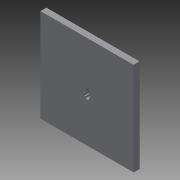
# Autodesk Inventor part: screwlockgen
Saved by Autodesk Inventor 2014 (Build 180170000, 170)
## iProperties
Created: 2014-07-13
Part Number: screwlockgen
Material: Generic
Document SubType Name: Modeling
Designer: cruiser
Density: 1 g/cm^3
Appearance: Default
Author: cruiser
Autodesk Inventor part; units mm, degrees
ref_plane "YZ Plane" through (0, 0, 0) normal (1, 0, 0) x (0, 1, 0)
ref_plane "XZ Plane" through (0, 0, 0) normal (0, 1, 0) x (-1, 0, 0)
ref_plane "XY Plane" through (0, 0, 0) normal (0, 0, 1) x (1, 0, 0)
sketch "Sketch1" plane through (0, 0, 0) normal (0, 1, 0) x (-1, 0, 0)
  line L0 (50, -50) -> (-50, -50)
  line L1 (-50, -50) -> (-50, 50)
  line L2 (-50, 50) -> (50, 50)
  line L3 (50, 50) -> (50, -50)
  line L4 (50, -50) -> (-50, 50) construction
  line L5 (-50, -50) -> (50, 50) construction
  point P0 (0, 0)
  dimension "d0" = 100
  dimension "d1" = 100
  constraints: 12 end point, 2 midpoint, 2 parallel, 1 horizontal, 1 perpendicular
  measures "d0" distance of L1.end L2.end
  measures "d1" distance of L0.end L1.end
extrude "Extrusion1" add sketch "Sketch1" along normal blind 6.35
sketch "Sketch7" plane through (0, 0, 0) normal (0, -1, 0) x (1, 0, 0)
  line L0 (1.65, -3.55) -> (-1.65, -3.55)
  line L1 (-1.65, -3.55) -> (-1.65, 3.55)
  line L2 (-1.65, 3.55) -> (1.65, 3.55)
  line L3 (1.65, 3.55) -> (1.65, -3.55)
  line L4 (1.65, -3.55) -> (-1.65, 3.55) construction
  line L5 (-1.65, -3.55) -> (1.65, 3.55) construction
  line L6 (2.75, -5.05) -> (-2.75, -5.05)
  line L7 (-2.75, -5.05) -> (-2.75, -2.05)
  line L8 (-2.75, -2.05) -> (2.75, -2.05)
  line L9 (2.75, -2.05) -> (2.75, -5.05)
  line L10 (2.75, -5.05) -> (-2.75, -2.05) construction
  line L11 (-2.75, -5.05) -> (2.75, -2.05) construction
  circle A0 centre (-2.75, -2.05) radius 0.5
  circle A1 centre (2.75, -2.05) radius 0.5
  circle A2 centre (2.75, -5.05) radius 0.5
  circle A3 centre (-2.75, -5.05) radius 0.5
  line L12 (-1.65, -3.55) -> (1.65, -3.55)
  line L13 (1.65, -3.55) -> (1.65, -5.05)
  line L14 (1.65, -5.05) -> (-1.65, -5.05)
  line L15 (-1.65, -5.05) -> (-1.65, -3.55)
  line L16 (-1.65, -5.05) -> (1.65, -5.05)
  line L17 (1.65, -5.05) -> (1.65, -7.05)
  line L18 (1.65, -7.05) -> (-1.65, -7.05)
  line L19 (-1.65, -7.05) -> (-1.65, -5.05)
  point P0 (0, 0)
  point P1 (0, -3.55)
  dimension "d49" = 8.6
  dimension "d50" = 3.3
  dimension "d51" = 5.5
  dimension "d52" = 3
  dimension "d55" = 1
  dimension "d56" = 1
  dimension "d57" = 1
  dimension "d58" = 1
  dimension "d59" = 2
  constraints: 40 end point, 8 parallel, 5 midpoint, 4 centre point, 4 coincident, 4 horizontal, 4 perpendicular, 2 collinear, 1 point on line
  measures "d49" distance between parallel lines of L6 L2
  measures "d50" distance between parallel lines of L3 L1
  measures "d51" distance between parallel lines of L7 L9
  measures "d52" distance between parallel lines of L6 L8
  measures "d55" diameter of A0
  measures "d56" diameter of A3
  measures "d57" diameter of A1
  measures "d58" diameter of A2
  measures "d59" distance between parallel lines of L6 L18
extrude "Extrusion7" cut sketch "Sketch7" against normal up to next
sketch "Sketch6" plane through (0, 0, 0) normal (0, -1, 0) x (1, 0, 0)
  line L0 (-50, -50) -> (50, -50) projected
  line L1 (50, 50) -> (-50, 50) projected
  line L2 (1.65, 42.9) -> (-1.65, 42.9)
  line L3 (-1.65, 42.9) -> (-1.65, 50)
  line L4 (-1.65, 50) -> (1.65, 50)
  line L5 (1.65, 50) -> (1.65, 42.9)
  line L6 (1.65, 42.9) -> (-1.65, 50) construction
  line L7 (-1.65, 42.9) -> (1.65, 50) construction
  line L8 (2.75, 41.4) -> (-2.75, 41.4)
  line L9 (-2.75, 41.4) -> (-2.75, 44.4)
  line L10 (-2.75, 44.4) -> (2.75, 44.4)
  line L11 (2.75, 44.4) -> (2.75, 41.4)
  line L12 (2.75, 41.4) -> (-2.75, 44.4) construction
  line L13 (-2.75, 41.4) -> (2.75, 44.4) construction
  line L14 (20.8795, -41.4) -> (-20.8795, -41.4)
  line L15 (-20.8795, -41.4) -> (-20.8795, 41.4)
  line L16 (-20.8795, 41.4) -> (20.8795, 41.4)
  line L17 (20.8795, 41.4) -> (20.8795, -41.4)
  line L18 (20.8795, -41.4) -> (-20.8795, 41.4) construction
  line L19 (-20.8795, -41.4) -> (20.8795, 41.4) construction
  line L20 (0, 41.4) -> (0, -41.4)
  point P0 (0, 0)
  point P1 (0, 46.45)
  point P2 (0, 42.9)
  dimension "d43" = 8.6
  dimension "d44" = 3
  dimension "d45" = 5.5
  dimension "d46" = 3.3
  constraints: 38 end point, 9 midpoint, 7 parallel, 3 perpendicular, 2 collinear, 2 horizontal, 1 other
  measures "d43" distance between parallel lines of L1 L16
  measures "d44" distance between parallel lines of L16 L10
  measures "d45" distance between parallel lines of L11 L9
  measures "d46" distance between parallel lines of L3 L5
sketch "Sketch5" plane through (0, 6.35, 0) normal (0, 1, 0) x (1, 0, 0)
  line L0 (50, 50) -> (-50, 50) projected
  line L1 (1.65, 50) -> (0, 50)
  line L2 (0, 50) -> (0, 0)
  line L3 (0, 0) -> (1.65, 0)
  line L4 (1.65, 0) -> (1.65, 50)
  line L5 (0, 0) -> (-1.65, 0)
  line L6 (-1.65, 0) -> (-1.65, 50)
  line L7 (-1.65, 50) -> (0, 50)
  line L8 (0, 50) -> (0, 0)
  line L9 (-1.65, 41.4) -> (1.65, 41.4)
  line L10 (2.75, 41.4) -> (-2.75, 41.4)
  line L11 (-2.75, 41.4) -> (-2.75, 44.4)
  line L12 (-2.75, 44.4) -> (2.75, 44.4)
  line L13 (2.75, 44.4) -> (2.75, 41.4)
  dimension "d36" = 3.3
  dimension "d37" = 8.6
  dimension "d38" = 5.5
  dimension "d39" = 3
  dimension "d40" = 0
  constraints: 26 end point, 6 parallel, 4 perpendicular, 4 point on line, 3 horizontal, 2 other
  measures "d36" distance between parallel lines of L4 L6
  measures "d37" distance between parallel lines of L9 L0
  measures "d38" distance between parallel lines of L13 L11
  measures "d39" distance between parallel lines of L12 L10
  measures "d40" distance between parallel lines of L9 L10
equation "\"d49\" = screw_length - m2_thickness"
equation "\"d50\" = screw_width"
equation "\"d51\" = nut_width"
equation "\"d52\" = nut_thickness"
equation "\"d55\" = relief"
equation "\"d56\" = relief"
equation "\"d57\" = relief"
equation "\"d58\" = relief"
equation "\"d59\" = extra_screw"
equation "\"d43\" = screw_length - m2_thickness"
equation "\"d44\" = nut_thickness"
equation "\"d45\" = nut_width"
equation "\"d46\" = screw_width"
equation "\"d36\" = screw_width"
equation "\"d37\" = screw_length - m2_thickness"
equation "\"d38\" = nut_width"
equation "\"d39\" = nut_thickness"
equation "\"m2_thickness\" = 6.4"
equation "\"screw_length\" = 15"
equation "\"nut_width\" = 5.5"
equation "\"nut_thickness\" = 3"
equation "\"screw_width\" = 3.3"
equation "\"relief\" = 1"
equation "\"extra_screw\" = 2"
body "Solid1"
